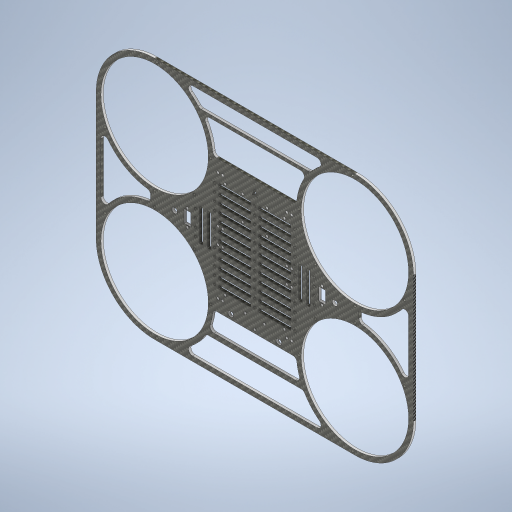
# Autodesk Inventor part: v3_top_carbon_fiber
Saved by Autodesk Inventor 2024 (Build 280153000, 153)
## iProperties
Created: 2025-03-06
Part Number: v3_top_carbon_fiber
Material: Generic
Document SubType Name: Modeling
Designer: Bruno
Density: 1 g/cm^3
Appearance: Default
Author: Bruno
Autodesk Inventor part; units mm, degrees
ref_plane "YZ Plane" through (0, 0, 0) normal (1, 0, 0) x (0, 1, 0)
ref_plane "XZ Plane" through (0, 0, 0) normal (0, 1, 0) x (-1, 0, 0)
ref_plane "XY Plane" through (0, 0, 0) normal (0, 0, 1) x (1, 0, 0)
sketch "Sketch1" plane through (0, 0, 0) normal (0, 0, 1) x (1, 0, 0)
  line L0 (-125, 79) -> (125, 79)
  line L1 (-125, 79) -> (-125, -79)
  line L2 (-125, -79) -> (125, -79)
  line L3 (125, -79) -> (125, 79)
  line L4 (-239.9943, 0) -> (241.4628, 0)
  line L5 (0, 173.5298) -> (0, -169.5298)
  line L6 (52.1097, 83) -> (0, 83)
  line L7 (130, 6.1714) -> (130, 0)
  line L8 (198, 79) -> (198, 0)
  line L9 (125, 152) -> (0, 152)
  line L10 (52.1097, -83) -> (0, -83)
  line L11 (130, -6.1714) -> (130, 0)
  line L12 (198, -79) -> (198, 0)
  line L13 (125, -152) -> (0, -152)
  line L14 (125, 146) -> (0, 146)
  line L15 (192, 79) -> (192, 0)
  line L16 (125, -146) -> (0, -146)
  line L17 (192, -79) -> (192, 0)
  line L18 (-52.1097, 83) -> (0, 83)
  line L19 (-130, 6.1714) -> (-130, 0)
  line L20 (-198, 79) -> (-198, 0)
  line L21 (-125, 152) -> (0, 152)
  line L22 (-125, -152) -> (0, -152)
  line L23 (-52.1097, -83) -> (0, -83)
  line L24 (-198, -79) -> (-198, 0)
  line L25 (-130, -6.1714) -> (-130, 0)
  line L26 (-125, 146) -> (0, 146)
  line L27 (-192, 79) -> (-192, 0)
  line L28 (-125, -146) -> (0, -146)
  line L29 (-192, -79) -> (-192, 0)
  circle A0 centre (122.1995, 148.944) radius 1.5
  circle A1 centre (186.9735, 46.4534) radius 1.5
  circle A2 centre (125, 9) radius 1.5
  circle A3 centre (55, 79) radius 1.5
  circle A4 centre (75.5025, 29.5025) radius 1.5
  circle A5 centre (122.1995, -148.944) radius 1.5
  circle A6 centre (186.9735, -46.4534) radius 1.5
  circle A7 centre (125, -9) radius 1.5
  circle A8 centre (55, -79) radius 1.5
  circle A9 centre (75.5025, -29.5025) radius 1.5
  circle A10 centre (-122.1995, 148.944) radius 1.5
  circle A11 centre (-186.9735, 46.4534) radius 1.5
  circle A12 centre (-125, 9) radius 1.5
  circle A13 centre (-55, 79) radius 1.5
  circle A14 centre (-75.5025, 29.5025) radius 1.5
  circle A15 centre (-122.1995, -148.944) radius 1.5
  circle A16 centre (-55, -79) radius 1.5
  circle A17 centre (-75.5025, -29.5025) radius 1.5
  circle A18 centre (-125, -9) radius 1.5
  circle A19 centre (-186.9735, -46.4534) radius 1.5
  line L30 (-125, -79) -> (125, 79)
  line L31 (75.5025, 29.5025) -> (125, 79)
  line L32 (122.1995, 148.944) -> (125, 79)
  line L33 (125, 79) -> (186.9735, 46.4534)
  circle A20 centre (125, 79) radius 70
  circle A21 centre (125, 79) radius 67
  circle A22 centre (125, 79) radius 73
  circle A23 centre (125, -79) radius 67
  circle A24 centre (125, -79) radius 73
  circle A25 centre (-125, 79) radius 67
  circle A26 centre (-125, 79) radius 73
  circle A27 centre (-125, -79) radius 67
  circle A28 centre (-125, -79) radius 73
  point P0 (0, 0)
  point P1 (-125, 0)
  point P2 (125, 0)
  point P3 (0, 79)
  point P4 (0, 0)
  point P5 (52, 79)
  point P6 (-52, 79)
  point P7 (-96.0172, 146)
  point P8 (96.0172, 146)
  point P9 (192, 50.0172)
  point P10 (192, -50.0172)
  point P11 (130, -6.1714)
  point P12 (130, 7.4586)
  point P13 (96.0172, -146)
  point P14 (-96.0172, -146)
  point P15 (-52, -79)
  point P16 (52, -79)
  point P17 (-192, 50.0172)
  point P18 (-130, 6.1714)
  point P19 (-130, -6.1714)
  point P20 (-192, -50.0172)
  point P21 (-198, 79)
  point P22 (-198, -79)
  point P23 (-125, -152)
  point P24 (125, -152)
  point P25 (198, -79)
  dimension "d2" = 250
  dimension "d3" = 158
  dimension "d16" = 166
  dimension "d17" = 260
  dimension "d35" = 3
  dimension "d36" = 3
  dimension "d37" = 3
  dimension "d40" = 3
  dimension "d42" = 3
  dimension "d62" = 45
  dimension "d64" = 120
  dimension "d65" = 120
  dimension "d66" = 140
  dimension "d127" = 134
  dimension "d128" = 146
  constraints: 68 end point, 45 symmetric about line, 29 centre point, 11 point on circle, 11 point on line, 8 coincident, 7 perpendicular, 4 midpoint, 4 tangent, 3 horizontal, 1 vertical, 21 other
  measures "d2" distance of L0.start L0.end
  measures "d3" distance of L2.end L0.end
  measures "d16" diameter of L6 L4
  measures "d17" diameter of L7 L5
  measures "d35" diameter of A0
  measures "d36" diameter of A1
  measures "d37" diameter of A2
  measures "d40" diameter of A3
  measures "d42" diameter of A4
  measures "d62" angle of L0 L31
  measures "d64" angle of L30 L33
  measures "d65" angle of L30 L32
  measures "d66" diameter of A20
  measures "d127" diameter of A21
  measures "d128" diameter of A22
extrude "Extrusion1" add sketch "Sketch1" along normal blind 3 contours A25 L26 A26 L0 A13 | L0 A13 A26 L1 A12 A25 | L1 A12 A26 L27 A25 | A25 L27 A26 L26 | A26 L21 L5 L26 | L27 L4 L20 A26 | A26 L18 L5 L0 | L0 L5 L4 L1 A26 | L5 L9 A22 L14 | L1 L4 L19 A26 | L29 A28 L24 L4 | L5 L6 A22 L0 | L0 A22 L30 L5 | A22 L15 A20 A0 L14 | L14 A20 A3 L0 A22 | L4 L30 A28 L1 | L1 A28 L25 L4 | A28 L1 A18 A27 L29 | L29 A27 L28 A28 | L0 A3 A20 L30 A22 | L30 A22 L3 L4 | L4 L3 A24 L2 L5 | L5 L2 A28 L30 | A20 A0 L32 L14 | L14 L32 A21 L0 A3 A20 | A28 L30 A27 L1 A18 | L30 A20 A4 A2 L3 A22 | L4 L11 A24 L3 | L3 A22 L7 L4 | L5 L23 A28 L2 | L2 A24 L10 L5 | A28 L2 A16 A27 L30 | L8 L4 L15 A22 | L32 A0 A20 L15 A21 L14 | L14 A21 L32 | A28 L28 L5 L22 | A27 L2 A16 A28 L28 | A3 L0 A21 L30 A20 | L30 A21 L31 A4 A20 | L3 A2 A20 A1 L15 A22 | A24 L17 A23 L3 A7 | L3 A7 A23 L2 A8 A24 | L2 A8 A23 L16 A24 | L12 A24 L17 L4 | L5 L16 A24 L13 | A24 L16 A23 L17 | A20 A1 L33 A21 L15 | A21 L3 A2 A20 A4 L31 | L33 A1 A20 A2 L3 A21
fillet "Fillet1" radius 5 15 edges at (52.1097, 83, 1.5) (-52.1097, 83, 1.5) (-96.0172, 146, 1.5) (96.0172, 146, 1.5) (-52.1097, -83, 1.5) (52.1097, -83, 1.5) (-96.0172, -146, 1.5) (96.0172, -146, 1.5) (-192, 50.0172, 1.5) (-130, 6.1714, 1.5) (-130, -6.1714, 1.5) (-192, -50.0172, 1.5) (130, -6.1714, 1.5) (192, 50.0172, 1.5) (192, -50.0172, 1.5)
sketch "Sketch2" plane through (0, 0, 3) normal (0, 0, 1) x (1, 0, 0)
  line L0 (-257.4929, 0) -> (257.4929, 0)
  line L1 (0, 208.8663) -> (0, -208.8663)
  line L2 (-47.521, -83) -> (47.521, -83) projected
  line L3 (-44, -53) -> (-6, -53)
  line L4 (-5, -54) -> (-5, -56)
  line L5 (-6, -57) -> (-44, -57)
  line L6 (-45, -56) -> (-45, -54)
  arc A0 (-44, -53) -> (-45, -54) centre (-44, -54) ccw
  arc A1 (-45, -56) -> (-44, -57) centre (-44, -56) ccw
  arc A2 (-6, -57) -> (-5, -56) centre (-6, -56) ccw
  arc A3 (-5, -54) -> (-6, -53) centre (-6, -54) ccw
  line L7 (44, -53) -> (6, -53)
  line L8 (5, -54) -> (5, -56)
  line L9 (6, -57) -> (44, -57)
  line L10 (45, -56) -> (45, -54)
  arc A4 (45, -54) -> (44, -53) centre (44, -54) ccw
  arc A5 (44, -57) -> (45, -56) centre (44, -56) ccw
  arc A6 (5, -56) -> (6, -57) centre (6, -56) ccw
  arc A7 (6, -53) -> (5, -54) centre (6, -54) ccw
  line L11 (-69.9007, -55) -> (69.9007, -55)
  circle A8 centre (0, -55) radius 1.5
  circle A9 centre (-50, -55) radius 1.5
  circle A10 centre (50, -55) radius 1.5
  circle A11 centre (-50, -45) radius 1.5
  line L12 (-45, -46) -> (-45, -44)
  arc A12 (-44, -43) -> (-45, -44) centre (-44, -44) ccw
  line L13 (-44, -43) -> (-6, -43)
  arc A13 (-45, -46) -> (-44, -47) centre (-44, -46) ccw
  line L14 (-6, -47) -> (-44, -47)
  arc A14 (-5, -44) -> (-6, -43) centre (-6, -44) ccw
  line L15 (-5, -44) -> (-5, -46)
  arc A15 (-6, -47) -> (-5, -46) centre (-6, -46) ccw
  circle A16 centre (0, -45) radius 1.5
  arc A17 (6, -43) -> (5, -44) centre (6, -44) ccw
  line L16 (5, -44) -> (5, -46)
  line L17 (44, -43) -> (6, -43)
  arc A18 (5, -46) -> (6, -47) centre (6, -46) ccw
  line L18 (6, -47) -> (44, -47)
  circle A19 centre (50, -45) radius 1.5
  line L19 (45, -46) -> (45, -44)
  arc A20 (45, -44) -> (44, -43) centre (44, -44) ccw
  arc A21 (44, -47) -> (45, -46) centre (44, -46) ccw
  circle A22 centre (-50, -35) radius 1.5
  line L20 (-45, -36) -> (-45, -34)
  arc A23 (-44, -33) -> (-45, -34) centre (-44, -34) ccw
  line L21 (-44, -33) -> (-6, -33)
  arc A24 (-45, -36) -> (-44, -37) centre (-44, -36) ccw
  line L22 (-6, -37) -> (-44, -37)
  arc A25 (-5, -34) -> (-6, -33) centre (-6, -34) ccw
  line L23 (-5, -34) -> (-5, -36)
  arc A26 (-6, -37) -> (-5, -36) centre (-6, -36) ccw
  circle A27 centre (0, -35) radius 1.5
  arc A28 (6, -33) -> (5, -34) centre (6, -34) ccw
  line L24 (5, -34) -> (5, -36)
  line L25 (44, -33) -> (6, -33)
  arc A29 (5, -36) -> (6, -37) centre (6, -36) ccw
  line L26 (6, -37) -> (44, -37)
  circle A30 centre (50, -35) radius 1.5
  line L27 (45, -36) -> (45, -34)
  arc A31 (45, -34) -> (44, -33) centre (44, -34) ccw
  arc A32 (44, -37) -> (45, -36) centre (44, -36) ccw
  circle A33 centre (-50, -25) radius 1.5
  line L28 (-45, -26) -> (-45, -24)
  arc A34 (-44, -23) -> (-45, -24) centre (-44, -24) ccw
  line L29 (-44, -23) -> (-6, -23)
  arc A35 (-45, -26) -> (-44, -27) centre (-44, -26) ccw
  line L30 (-6, -27) -> (-44, -27)
  arc A36 (-5, -24) -> (-6, -23) centre (-6, -24) ccw
  line L31 (-5, -24) -> (-5, -26)
  arc A37 (-6, -27) -> (-5, -26) centre (-6, -26) ccw
  circle A38 centre (0, -25) radius 1.5
  arc A39 (6, -23) -> (5, -24) centre (6, -24) ccw
  line L32 (5, -24) -> (5, -26)
  line L33 (44, -23) -> (6, -23)
  arc A40 (5, -26) -> (6, -27) centre (6, -26) ccw
  line L34 (6, -27) -> (44, -27)
  circle A41 centre (50, -25) radius 1.5
  line L35 (45, -26) -> (45, -24)
  arc A42 (45, -24) -> (44, -23) centre (44, -24) ccw
  arc A43 (44, -27) -> (45, -26) centre (44, -26) ccw
  circle A44 centre (-50, -15) radius 1.5
  line L36 (-45, -16) -> (-45, -14)
  arc A45 (-44, -13) -> (-45, -14) centre (-44, -14) ccw
  line L37 (-44, -13) -> (-6, -13)
  arc A46 (-45, -16) -> (-44, -17) centre (-44, -16) ccw
  line L38 (-6, -17) -> (-44, -17)
  arc A47 (-5, -14) -> (-6, -13) centre (-6, -14) ccw
  line L39 (-5, -14) -> (-5, -16)
  arc A48 (-6, -17) -> (-5, -16) centre (-6, -16) ccw
  circle A49 centre (0, -15) radius 1.5
  arc A50 (6, -13) -> (5, -14) centre (6, -14) ccw
  line L40 (5, -14) -> (5, -16)
  line L41 (44, -13) -> (6, -13)
  arc A51 (5, -16) -> (6, -17) centre (6, -16) ccw
  line L42 (6, -17) -> (44, -17)
  circle A52 centre (50, -15) radius 1.5
  line L43 (45, -16) -> (45, -14)
  arc A53 (45, -14) -> (44, -13) centre (44, -14) ccw
  arc A54 (44, -17) -> (45, -16) centre (44, -16) ccw
  circle A55 centre (-50, -5) radius 1.5
  line L44 (-45, -6) -> (-45, -4)
  arc A56 (-44, -3) -> (-45, -4) centre (-44, -4) ccw
  line L45 (-44, -3) -> (-6, -3)
  arc A57 (-45, -6) -> (-44, -7) centre (-44, -6) ccw
  line L46 (-6, -7) -> (-44, -7)
  arc A58 (-5, -4) -> (-6, -3) centre (-6, -4) ccw
  line L47 (-5, -4) -> (-5, -6)
  arc A59 (-6, -7) -> (-5, -6) centre (-6, -6) ccw
  circle A60 centre (0, -5) radius 1.5
  arc A61 (6, -3) -> (5, -4) centre (6, -4) ccw
  line L48 (5, -4) -> (5, -6)
  line L49 (44, -3) -> (6, -3)
  arc A62 (5, -6) -> (6, -7) centre (6, -6) ccw
  line L50 (6, -7) -> (44, -7)
  circle A63 centre (50, -5) radius 1.5
  line L51 (45, -6) -> (45, -4)
  arc A64 (45, -4) -> (44, -3) centre (44, -4) ccw
  arc A65 (44, -7) -> (45, -6) centre (44, -6) ccw
  circle A66 centre (-50, 5) radius 1.5
  line L52 (-45, 4) -> (-45, 6)
  arc A67 (-44, 7) -> (-45, 6) centre (-44, 6) ccw
  line L53 (-44, 7) -> (-6, 7)
  arc A68 (-45, 4) -> (-44, 3) centre (-44, 4) ccw
  line L54 (-6, 3) -> (-44, 3)
  arc A69 (-5, 6) -> (-6, 7) centre (-6, 6) ccw
  line L55 (-5, 6) -> (-5, 4)
  arc A70 (-6, 3) -> (-5, 4) centre (-6, 4) ccw
  circle A71 centre (0, 5) radius 1.5
  arc A72 (6, 7) -> (5, 6) centre (6, 6) ccw
  line L56 (5, 6) -> (5, 4)
  line L57 (44, 7) -> (6, 7)
  arc A73 (5, 4) -> (6, 3) centre (6, 4) ccw
  line L58 (6, 3) -> (44, 3)
  circle A74 centre (50, 5) radius 1.5
  line L59 (45, 4) -> (45, 6)
  arc A75 (45, 6) -> (44, 7) centre (44, 6) ccw
  arc A76 (44, 3) -> (45, 4) centre (44, 4) ccw
  circle A77 centre (-50, 15) radius 1.5
  line L60 (-45, 14) -> (-45, 16)
  arc A78 (-44, 17) -> (-45, 16) centre (-44, 16) ccw
  line L61 (-44, 17) -> (-6, 17)
  arc A79 (-45, 14) -> (-44, 13) centre (-44, 14) ccw
  line L62 (-6, 13) -> (-44, 13)
  arc A80 (-5, 16) -> (-6, 17) centre (-6, 16) ccw
  line L63 (-5, 16) -> (-5, 14)
  arc A81 (-6, 13) -> (-5, 14) centre (-6, 14) ccw
  circle A82 centre (0, 15) radius 1.5
  arc A83 (6, 17) -> (5, 16) centre (6, 16) ccw
  line L64 (5, 16) -> (5, 14)
  line L65 (44, 17) -> (6, 17)
  arc A84 (5, 14) -> (6, 13) centre (6, 14) ccw
  line L66 (6, 13) -> (44, 13)
  circle A85 centre (50, 15) radius 1.5
  line L67 (45, 14) -> (45, 16)
  arc A86 (45, 16) -> (44, 17) centre (44, 16) ccw
  arc A87 (44, 13) -> (45, 14) centre (44, 14) ccw
  circle A88 centre (-50, 25) radius 1.5
  line L68 (-45, 24) -> (-45, 26)
  arc A89 (-44, 27) -> (-45, 26) centre (-44, 26) ccw
  line L69 (-44, 27) -> (-6, 27)
  arc A90 (-45, 24) -> (-44, 23) centre (-44, 24) ccw
  line L70 (-6, 23) -> (-44, 23)
  arc A91 (-5, 26) -> (-6, 27) centre (-6, 26) ccw
  line L71 (-5, 26) -> (-5, 24)
  arc A92 (-6, 23) -> (-5, 24) centre (-6, 24) ccw
  circle A93 centre (0, 25) radius 1.5
  arc A94 (6, 27) -> (5, 26) centre (6, 26) ccw
  line L72 (5, 26) -> (5, 24)
  line L73 (44, 27) -> (6, 27)
  arc A95 (5, 24) -> (6, 23) centre (6, 24) ccw
  line L74 (6, 23) -> (44, 23)
  circle A96 centre (50, 25) radius 1.5
  line L75 (45, 24) -> (45, 26)
  arc A97 (45, 26) -> (44, 27) centre (44, 26) ccw
  arc A98 (44, 23) -> (45, 24) centre (44, 24) ccw
  circle A99 centre (-50, 35) radius 1.5
  line L76 (-45, 34) -> (-45, 36)
  arc A100 (-44, 37) -> (-45, 36) centre (-44, 36) ccw
  line L77 (-44, 37) -> (-6, 37)
  arc A101 (-45, 34) -> (-44, 33) centre (-44, 34) ccw
  line L78 (-6, 33) -> (-44, 33)
  arc A102 (-5, 36) -> (-6, 37) centre (-6, 36) ccw
  line L79 (-5, 36) -> (-5, 34)
  arc A103 (-6, 33) -> (-5, 34) centre (-6, 34) ccw
  circle A104 centre (0, 35) radius 1.5
  arc A105 (6, 37) -> (5, 36) centre (6, 36) ccw
  line L80 (5, 36) -> (5, 34)
  line L81 (44, 37) -> (6, 37)
  arc A106 (5, 34) -> (6, 33) centre (6, 34) ccw
  line L82 (6, 33) -> (44, 33)
  circle A107 centre (50, 35) radius 1.5
  line L83 (45, 34) -> (45, 36)
  arc A108 (45, 36) -> (44, 37) centre (44, 36) ccw
  arc A109 (44, 33) -> (45, 34) centre (44, 34) ccw
  circle A110 centre (-50, 45) radius 1.5
  line L84 (-45, 44) -> (-45, 46)
  arc A111 (-44, 47) -> (-45, 46) centre (-44, 46) ccw
  line L85 (-44, 47) -> (-6, 47)
  arc A112 (-45, 44) -> (-44, 43) centre (-44, 44) ccw
  line L86 (-6, 43) -> (-44, 43)
  arc A113 (-5, 46) -> (-6, 47) centre (-6, 46) ccw
  line L87 (-5, 46) -> (-5, 44)
  arc A114 (-6, 43) -> (-5, 44) centre (-6, 44) ccw
  circle A115 centre (0, 45) radius 1.5
  arc A116 (6, 47) -> (5, 46) centre (6, 46) ccw
  line L88 (5, 46) -> (5, 44)
  line L89 (44, 47) -> (6, 47)
  arc A117 (5, 44) -> (6, 43) centre (6, 44) ccw
  line L90 (6, 43) -> (44, 43)
  circle A118 centre (50, 45) radius 1.5
  line L91 (45, 44) -> (45, 46)
  arc A119 (45, 46) -> (44, 47) centre (44, 46) ccw
  arc A120 (44, 43) -> (45, 44) centre (44, 44) ccw
  circle A121 centre (-50, 55) radius 1.5
  line L92 (-45, 54) -> (-45, 56)
  arc A122 (-44, 57) -> (-45, 56) centre (-44, 56) ccw
  line L93 (-44, 57) -> (-6, 57)
  arc A123 (-45, 54) -> (-44, 53) centre (-44, 54) ccw
  line L94 (-6, 53) -> (-44, 53)
  arc A124 (-5, 56) -> (-6, 57) centre (-6, 56) ccw
  line L95 (-5, 56) -> (-5, 54)
  arc A125 (-6, 53) -> (-5, 54) centre (-6, 54) ccw
  circle A126 centre (0, 55) radius 1.5
  arc A127 (6, 57) -> (5, 56) centre (6, 56) ccw
  line L96 (5, 56) -> (5, 54)
  line L97 (44, 57) -> (6, 57)
  arc A128 (5, 54) -> (6, 53) centre (6, 54) ccw
  line L98 (6, 53) -> (44, 53)
  circle A129 centre (50, 55) radius 1.5
  line L99 (45, 54) -> (45, 56)
  arc A130 (45, 56) -> (44, 57) centre (44, 56) ccw
  arc A131 (44, 53) -> (45, 54) centre (44, 54) ccw
  line L100 (0, 73) -> (-3.5, 65)
  line L101 (-3.5, 65) -> (0, 67)
  line L102 (0, 73) -> (3.5, 65)
  line L103 (3.5, 65) -> (0, 67)
  line L104 (-62, 18.8087) -> (-62, -18.8087)
  line L105 (-58, 20) -> (-56, 20)
  line L106 (-55, 19) -> (-55, -19)
  line L107 (-56, -20) -> (-58, -20)
  line L108 (-59, -19) -> (-59, 19)
  line L109 (-66, 20) -> (-68, 20)
  line L110 (-69, 19) -> (-69, -19)
  line L111 (-68, -20) -> (-66, -20)
  line L112 (-65, -19) -> (-65, 19)
  circle A132 centre (-74, -15) radius 1.5
  circle A133 centre (-74, -5) radius 1.5
  circle A134 centre (-74, 5) radius 1.5
  circle A135 centre (-74, 15) radius 1.5
  line L113 (58, 20) -> (56, 20)
  line L114 (55, 19) -> (55, -19)
  line L115 (56, -20) -> (58, -20)
  line L116 (59, -19) -> (59, 19)
  line L117 (66, 20) -> (68, 20)
  line L118 (65, -19) -> (65, 19)
  line L119 (69, 19) -> (69, -19)
  line L120 (68, -20) -> (66, -20)
  circle A136 centre (74, 15) radius 1.5
  circle A137 centre (74, 5) radius 1.5
  circle A138 centre (74, -5) radius 1.5
  circle A139 centre (74, -15) radius 1.5
  arc A140 (-68, 20) -> (-69, 19) centre (-68, 19) ccw
  arc A141 (-65, 19) -> (-66, 20) centre (-66, 19) ccw
  arc A142 (-66, -20) -> (-65, -19) centre (-66, -19) ccw
  arc A143 (-69, -19) -> (-68, -20) centre (-68, -19) ccw
  arc A144 (-56, -20) -> (-55, -19) centre (-56, -19) ccw
  arc A145 (-59, -19) -> (-58, -20) centre (-58, -19) ccw
  arc A146 (-58, 20) -> (-59, 19) centre (-58, 19) ccw
  arc A147 (-55, 19) -> (-56, 20) centre (-56, 19) ccw
  arc A148 (56, 20) -> (55, 19) centre (56, 19) ccw
  arc A149 (59, 19) -> (58, 20) centre (58, 19) ccw
  arc A150 (66, 20) -> (65, 19) centre (66, 19) ccw
  arc A151 (69, 19) -> (68, 20) centre (68, 19) ccw
  arc A152 (55, -19) -> (56, -20) centre (56, -19) ccw
  arc A153 (58, -20) -> (59, -19) centre (58, -19) ccw
  arc A154 (65, -19) -> (66, -20) centre (66, -19) ccw
  arc A155 (68, -20) -> (69, -19) centre (68, -19) ccw
  line L121 (-46, -10) -> (46, -10)
  line L122 (46, -10) -> (46, -68)
  line L123 (46, -68) -> (-46, -68)
  line L124 (-46, -68) -> (-46, -10)
  circle A156 centre (-46, -68) radius 1.5
  circle A157 centre (-40, -68) radius 1.5
  line L125 (-46, -39) -> (46, -39)
  circle A158 centre (46, -68) radius 1.5
  circle A159 centre (40, -68) radius 1.5
  circle A160 centre (-46, -10) radius 1.5
  circle A161 centre (-40, -10) radius 1.5
  circle A162 centre (46, -10) radius 1.5
  circle A163 centre (40, -10) radius 1.5
  circle A164 centre (-46, 68) radius 1.5
  circle A165 centre (-40, 68) radius 1.5
  circle A166 centre (46, 68) radius 1.5
  circle A167 centre (40, 68) radius 1.5
  circle A168 centre (-46, 10) radius 1.5
  circle A169 centre (-40, 10) radius 1.5
  circle A170 centre (40, 10) radius 1.5
  circle A171 centre (46, 10) radius 1.5
  circle A172 centre (-100, 0) radius 3.25
  line L126 (-101.7321, 2.75) -> (-98.2679, 2.75)
  circle A173 centre (100, 0) radius 3.25
  line L127 (101.7321, 2.75) -> (98.2679, 2.75)
  circle A174 centre (-30, -77) radius 3.25
  line L128 (-31.7321, -74.25) -> (-28.2679, -74.25)
  circle A175 centre (30, -77) radius 3.25
  line L129 (31.7321, -74.25) -> (28.2679, -74.25)
  line L130 (-15.7268, -67) -> (15.7268, -67)
  circle A176 centre (-12, -67) radius 1.5
  circle A177 centre (12, -67) radius 1.5
  circle A178 centre (0, -79) radius 1.5
  line L131 (-88.1, 7.8) -> (-80, 7.8)
  line L132 (-80, 7.8) -> (-80, -7.8)
  line L133 (-80, -7.8) -> (-88.1, -7.8)
  line L134 (-88.1, -7.8) -> (-88.1, 7.8)
  line L135 (-84.05, 20.75) -> (-84.05, -20.75)
  circle A179 centre (-84.05, 10.25) radius 1.5
  circle A180 centre (-84.05, -10.25) radius 1.5
  line L136 (88.1, 7.8) -> (80, 7.8)
  line L137 (80, 7.8) -> (80, -7.8)
  line L138 (80, -7.8) -> (88.1, -7.8)
  line L139 (88.1, -7.8) -> (88.1, 7.8)
  circle A181 centre (84.05, 10.25) radius 1.5
  circle A182 centre (84.05, -10.25) radius 1.5
  line L140 (-24.9023, 45) -> (24.9023, 45)
  circle A183 centre (-15.25, 60.25) radius 1.5
  circle A184 centre (-15.25, 29.75) radius 1.5
  circle A185 centre (15.25, 60.25) radius 1.5
  circle A186 centre (15.25, 29.75) radius 1.5
  circle A187 centre (-37, -60) radius 1.5
  circle A188 centre (37, -60) radius 1.5
  line L141 (-83.4003, 0) -> (83.4003, 0)
  circle A189 centre (-37, 60) radius 1.5
  circle A190 centre (37, 60) radius 1.5
  point P0 (0, 0)
  point P1 (0, 0)
  point P2 (-47.1508, -83)
  point P3 (47.1508, -83)
  point P4 (-5, -57)
  point P5 (-5, -53)
  point P6 (-45, -57)
  point P7 (-45, -55)
  point P8 (-45, -47)
  point P9 (-45, -45)
  point P10 (-5, -43)
  point P11 (-5, -47)
  point P12 (-45, -37)
  point P13 (-45, -35)
  point P14 (-5, -33)
  point P15 (-5, -37)
  point P16 (-45, -27)
  point P17 (-45, -25)
  point P18 (-5, -23)
  point P19 (-5, -27)
  point P20 (-45, -17)
  point P21 (-45, -15)
  point P22 (-5, -13)
  point P23 (-5, -17)
  point P24 (-45, -7)
  point P25 (-45, -5)
  point P26 (-5, -3)
  point P27 (-5, -7)
  point P28 (-45, 3)
  point P29 (-45, 5)
  point P30 (-5, 7)
  point P31 (-5, 3)
  point P32 (-45, 13)
  point P33 (-45, 15)
  point P34 (-5, 17)
  point P35 (-5, 13)
  point P36 (-45, 23)
  point P37 (-45, 25)
  point P38 (-5, 27)
  point P39 (-5, 23)
  point P40 (-45, 33)
  point P41 (-45, 35)
  point P42 (-5, 37)
  point P43 (-5, 33)
  point P44 (-45, 43)
  point P45 (-45, 45)
  point P46 (-5, 47)
  point P47 (-5, 43)
  point P48 (-45, 53)
  point P49 (-45, 55)
  point P50 (-5, 57)
  point P51 (-5, 53)
  point P52 (-62, 0)
  point P53 (-59, 20)
  point P54 (-55, -20)
  point P55 (-55, 20)
  point P56 (-59, -20)
  point P57 (-55, 0)
  point P58 (-65, 20)
  point P59 (-69, -20)
  point P60 (-69, 20)
  point P61 (-65, -20)
  point P62 (59, 20)
  point P63 (55, -20)
  point P64 (55, 20)
  point P65 (59, -20)
  point P66 (65, 20)
  point P67 (69, 20)
  point P68 (65, -20)
  point P69 (69, -20)
  point P70 (0, -10)
  point P71 (0, -67)
  point P72 (-84.05, 7.8)
  point P73 (-84.05, 0)
  point P74 (-80, 0)
  point P75 (-52.2576, -83)
  point P76 (52.2576, -83)
  point P77 (0, 45)
  point P78 (0, 0)
  dimension "d67" = 4
  dimension "d68" = 10
  dimension "d69" = 40
  dimension "d72" = 1
  dimension "d73" = 3
  dimension "d74" = 3
  dimension "d78" = 10
  dimension "d83" = 6
  dimension "d84" = 100
  dimension "d85" = 10
  dimension "d87" = 7
  dimension "d88" = 6
  dimension "d89" = 8
  dimension "d90" = 62
  dimension "d91" = 4
  dimension "d92" = 6
  dimension "d93" = 40
  dimension "d94" = 1
  dimension "d95" = 15
  dimension "d96" = 58
  dimension "d97" = 92
  dimension "d98" = 3
  dimension "d99" = 3
  dimension "d100" = 6
  dimension "d108" = 6.5
  dimension "d109" = 200
  dimension "d110" = 6
  dimension "d111" = 6.5
  dimension "d112" = 6
  dimension "d113" = 60
  dimension "d114" = 6
  dimension "d115" = 3
  dimension "d116" = 12
  dimension "d119" = 3
  dimension "d120" = 24
  dimension "d121" = 24
  dimension "d122" = 8.1
  dimension "d123" = 15.6
  dimension "d124" = 160
  dimension "d125" = 3
  dimension "d126" = 20.5
  dimension "d130" = 45
  dimension "d131" = 3
  dimension "d132" = 30.5
  dimension "d133" = 30.5
  dimension "d141" = 74
  dimension "d142" = 3
  dimension "d144" = 120
  constraints: 341 vertical alignment, 280 end point, 232 point on circle, 191 centre point, 158 equal radius, 115 point on line, 54 parallel, 45 collinear, 44 horizontal alignment, 40 tangent, 24 symmetric about line, 14 midpoint, 9 horizontal, 4 perpendicular, 3 coincident, 2 vertical, 32 other
  measures "d67" distance of point (-5, -53) point (-5, -57)
  measures "d69" distance of point (-5, -57) point (-45, -57)
  measures "d72" radius of A0
  measures "d73" diameter of A8
  measures "d74" diameter of A9
  measures "d78" distance of A9.centre A11.centre
  measures "d83" diameter of L54 L0
  measures "d85" distance from line of L97 L101.end
  measures "d88" distance of L101.end L100.start
  measures "d89" vertical distance of L100.start L100.end
  measures "d90" distance of the line from the sketch origin of L104
  measures "d91" distance of point (-59, 20) point (-55, 20)
  measures "d92" distance between parallel lines of L108 L112
  measures "d93" distance of point (-55, 20) point (-55, -20)
  measures "d94" radius of A140
  measures "d95" distance from line of L2 L123.end
  measures "d96" distance of L123.end L121.start
  measures "d97" distance of L122.end L123.end
  measures "d98" diameter of A157
  measures "d99" diameter of A156
  measures "d100" distance of L123.end A157.centre
  measures "d108" diameter of A172
  measures "d111" diameter of A174
  measures "d114" distance from line of L2 A174.centre
  measures "d115" diameter of A176
  measures "d116" distance of point (0, -67) A176.centre
  measures "d119" diameter of A178
  measures "d120" diameter of A178.centre L130
  measures "d121" diameter of point (0, -55) L130
  measures "d122" distance of L131.start L131.end
  measures "d123" distance of L131.end L132.end
  measures "d125" diameter of A179
  measures "d126" diameter of A179.centre L0
  measures "d130" distance between parallel lines of L0 L140
  measures "d131" diameter of A183
  measures "d132" diameter of A183.centre L140
  measures "d142" diameter of A187
  measures "d144" diameter of A187.centre L141
extrude "Extrusion2" cut sketch "Sketch2" against normal through all contours A172 L126 L0 | A179 L135 | L135 A179 | L87 A114 L86 A112 L84 A111 L85 A113 | L101 L100 L1 | L1 L102 L103 | A126 L1 | L1 A126 | L88 A116 L89 A119 L91 A120 L90 A117 | A115 L140 L1 | L1 L140 A115 | A104 L1 | L1 A104 | A93 L1 | L1 A93 | A82 L1 | L1 A82 | A71 L1 | L1 A71 | A173 L127 L0 | L0 A173 | L137 L136 L139 L0 | L0 L139 L138 L137 | L118 A150 L117 A151 L119 L0 | L0 L119 A155 L120 A154 L118 | L114 A148 L113 A149 L116 L0 | L0 L116 A153 L115 A152 L114 | A10 L11 | L11 A10 | A178 L1 | L1 A178 | A9 L11 | L11 A9 | A60 L1 | L1 A60 | L108 A146 L105 A147 L106 L0 | L0 L106 A144 L107 A145 L108 | L110 A140 L109 A141 L112 L0 | L0 L112 A142 L111 A143 L110 | A180 L135 | L135 A180 | L134 L131 L135 L0 | L0 L135 L133 L134 | L0 A172 | L135 L131 L132 L0 | L0 L132 L133 L135 | A49 L1 | L1 A49 | A161 L121 | L121 A161 | A163 L121 | L121 A163 | A38 L1 | L1 A38 | A160 L124 L121 | L121 L124 A160 | A162 L122 L121 | L121 L122 A162 | A27 L1 | L1 A27 | L140 A115 L1 | L1 A115 L140 | L11 L4 A2 L5 A1 L6 | L6 A0 L3 A3 L4 L11 | A156 L123 L124 | L124 L123 A156 | A16 L1 | L1 A16 | L11 L8 A7 L7 A4 L10 | L10 A5 L9 A6 L8 L11 | A158 L123 L122 | L122 L123 A158 | A8 L1 L11 | L11 L1 A8 | A157 L123 | L123 A157 | A8 L11 L1 | A8 L1 L11 | A159 L123 | L123 A159 | A176 L130 L123 | L123 A176 | A177 L123 | L123 A177 L130 | L130 A176 | A177 L130 | A11 | L12 A12 L13 A14 L15 A15 L14 A13 | L17 A20 L19 A21 L18 A18 L16 A17 | A19 | A22 | L20 A23 L21 A25 L23 A26 L22 A24 | L25 A31 L27 A32 L26 A29 L24 A28 | A30 | A33 | L28 A34 L29 A36 L31 A37 L30 A35 | L33 A42 L35 A43 L34 A40 L32 A39 | A41 | A44 | L36 A45 L37 A47 L39 A48 L38 A46 | L41 A53 L43 A54 L42 A51 L40 A50 | A52 | A55 | L44 A56 L45 A58 L47 A59 L46 A57 | L49 A64 L51 A65 L50 A62 L48 A61 | A63 | A66 | L52 A67 L53 A69 L55 A70 L54 A68 | L57 A75 L59 A76 L58 A73 L56 A72 | A74 | A77 | L60 A78 L61 A80 L63 A81 L62 A79 | L65 A86 L67 A87 L66 A84 L64 A83 | A85 | A88 | L68 A89 L69 A91 L71 A92 L70 A90 | L73 A97 L75 A98 L74 A95 L72 A94 | A96 | A99 | L76 A100 L77 A102 L79 A103 L78 A101 | L81 A108 L83 A109 L82 A106 L80 A105 | A107 | A110 | A118 | A121 | L92 A122 L93 A124 L95 A125 L94 A123 | L97 A130 L99 A131 L98 A128 L96 A127 | A129 | A132 | A133 | A134 | A135 | A136 | A137 | A138 | A139 | A164 | A165 | A166 | A167 | A168 | A169 | A170 | A171 | A174 L128 | A175 L129 | A181 | A182 | A183 | A184 | A185 | A186 | A187 | A188 | A189 | A190 picked at (-30.526, -76.5114) picked at (30.959, -77.519)
sketch "Sketch6" plane through (0, 0, 3) normal (0, 0, 1) x (1, 0, 0)
  line L0 (-77.6714, 146) -> (77.6714, 146) projected
  arc A0 (-52.4876, 87.4231) -> (-80.7052, 137.0256) centre (-125, 79) ccw projected
  arc A1 (80.7052, 137.0256) -> (52.4876, 87.4231) centre (125, 79) ccw projected
  line L1 (47.521, 83) -> (-47.521, 83) projected
  line L2 (-47.521, -83) -> (47.521, -83) projected
  arc A2 (-80.7052, -137.0256) -> (-52.4876, -87.4231) centre (-125, -79) ccw projected
  line L3 (77.6714, -146) -> (-77.6714, -146) projected
  arc A3 (52.4876, -87.4231) -> (80.7052, -137.0256) centre (125, -79) ccw projected
  line L4 (-69.143, 126) -> (69.143, 126)
  line L5 (-66.0085, 122) -> (66.0085, 122)
  line L6 (-58.0075, -108) -> (58.0075, -108)
  line L7 (-60.9375, -114) -> (60.9375, -114)
  point P0 (0, 0)
  dimension "d135" = 6
  dimension "d136" = 25
  dimension "d137" = 20
  dimension "d138" = 4
  constraints: 8 end point, 8 point on circle, 2 horizontal, 2 parallel
  measures "d135" distance between parallel lines of L7 L6
  measures "d136" distance between parallel lines of L2 L6
  measures "d137" distance between parallel lines of L0 L4
  measures "d138" distance between parallel lines of L5 L4
extrude "Extrusion5" add sketch "Sketch6" against normal up to surface (3 mm away)
fillet "Fillet5" radius 5 8 edges at (66.0085, 122, 1.5) (69.143, 126, 1.5) (-69.143, 126, 1.5) (-66.0085, 122, 1.5) (-60.9375, -114, 1.5) (-58.0075, -108, 1.5) (60.9375, -114, 1.5) (58.0075, -108, 1.5)
sketch "Sketch3" plane through (0, 0, 0) normal (0, 0, -1) x (-1, 0, 0)
  line L0 (124, -100) -> (-124, -100)
  line L1 (-124, -100) -> (-124, 100)
  line L2 (-124, 100) -> (124, 100)
  line L3 (124, 100) -> (124, -100)
  line L4 (124, -100) -> (-124, 100)
  line L5 (204, -160) -> (-204, -160)
  line L6 (-204, -160) -> (-204, 160)
  line L7 (-204, 160) -> (204, 160)
  line L8 (204, 160) -> (204, -160)
  line L9 (-204, -160) -> (204, 160)
  point P0 (0, 0)
  point P1 (0, 0)
  dimension "d56" = 200
  dimension "d57" = 248
  dimension "d58" = 60
  dimension "d59" = 80
  constraints: 20 end point, 4 parallel, 2 horizontal, 2 midpoint, 2 perpendicular, 1 coincident
  measures "d56" distance of L2.end L0.start
  measures "d57" distance of L0.start L0.end
  measures "d58" distance between parallel lines of L0 L5
  measures "d59" distance between parallel lines of L8 L3
body "Solid1"
